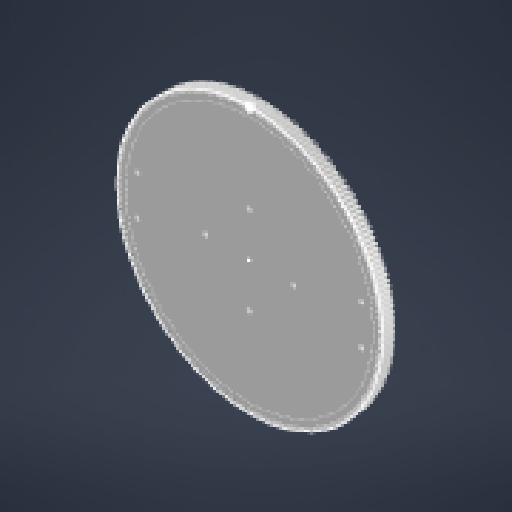
# Autodesk Inventor part: vertical_axis_bigl_gear
Saved by Autodesk Inventor 2023.2 (Build 272271000, 271)
## iProperties
Created: 2020-10-03
Part Number: vertical_axis_bigl_gear
Material: Generic
Document SubType Name: Modeling
Designer: bober
Density: 1 g/cm^3
Appearance: Default
Author: bober
Autodesk Inventor part; units mm, degrees
ref_plane "YZ Plane" through (0, 0, 0) normal (1, 0, 0) x (0, 1, 0)
ref_plane "XZ Plane" through (0, 0, 0) normal (0, 1, 0) x (-1, 0, 0)
ref_plane "XY Plane" through (0, 0, 0) normal (0, 0, 1) x (1, 0, 0)
sketch "Sketch1" plane through (0, 0, 0) normal (0, 0, 1) x (1, 0, 0)
  spline S0 degree 3 poles (-1.2656, 100.9921) (-1.1744, 100.7653) (-0.9921, 100.3117) (-0.7787, 99.7392) (-0.6166, 99.278) (-0.5147, 98.9901) (-0.458, 98.7994) (-0.4209, 98.7155) (-0.3986, 98.6754) (-0.3711, 98.6386) (-0.3402, 98.6046) (-0.3051, 98.575) (-0.267, 98.5494) (-0.2257, 98.5291) (-0.1823, 98.5143) (-0.1375, 98.5042) (-0.0764, 98.5001) (0, 98.5024) (0.0764, 98.5001) (0.1375, 98.5042) (0.1823, 98.5143) (0.2257, 98.5291) (0.267, 98.5494) (0.3051, 98.575) (0.3402, 98.6046) (0.3711, 98.6386) (0.3986, 98.6754) (0.4209, 98.7155) (0.458, 98.7994) (0.5147, 98.9901) (0.6166, 99.278) (0.7787, 99.7392) (0.9921, 100.3117) (1.1744, 100.7653) (1.2656, 100.9921) knots 0 0 0 0 0.07332 0.14664 0.1833 0.219961 0.238288 0.242867 0.247449 0.252032 0.256612 0.261194 0.265775 0.270356 0.274938 0.279519 0.284099 0.293264 0.30243 0.307009 0.311591 0.316173 0.320754 0.325335 0.329917 0.334497 0.33908 0.343662 0.348241 0.366568 0.403229 0.439889 0.513209 0.586529 0.586529 0.586529 0.586529
  circle A0 centre (0, 0) radius 98.5015 construction
  circle A1 centre (0, 0) radius 93.9693 construction
  circle A2 centre (0, 0) radius 100 construction
  circle A3 centre (0, 0) radius 101
  point P0 (-0.995, 100.3106)
  point P1 (-0.7389, 99.6236)
  point P2 (-0.6165, 99.2781)
  point P3 (-0.4982, 98.931)
  point P4 (-0.4391, 98.7576)
  point P5 (-0.4203, 98.7158)
  point P6 (-0.3977, 98.6759)
  point P7 (-0.3705, 98.6391)
  point P8 (-0.3395, 98.6053)
  point P9 (-0.3046, 98.5756)
  point P10 (-0.2665, 98.5503)
  point P11 (-0.2254, 98.53)
  point P12 (-0.1821, 98.5151)
  point P13 (-0.1373, 98.5053)
  point P14 (-0.0917, 98.5016)
  point P15 (0, 98.5015)
  point P16 (0.0917, 98.5016)
  point P17 (0.1373, 98.5053)
  point P18 (0.1821, 98.5151)
  point P19 (0.2254, 98.53)
  point P20 (0.2665, 98.5503)
  point P21 (0.3046, 98.5756)
  point P22 (0.3395, 98.6053)
  point P23 (0.3705, 98.6391)
  point P24 (0.3977, 98.6759)
  point P25 (0.4203, 98.7158)
  point P26 (0.4391, 98.7576)
  point P27 (0.4982, 98.931)
  point P28 (0.6165, 99.2781)
  point P29 (0.7389, 99.6236)
  point P30 (0.995, 100.3106)
  constraints: 4 centre point, 2 point on circle, 71 other
extrude "Extrusion1" add sketch "Sketch1" against normal blind 10
extrude "Extrusion2" cut sketch "Sketch1" against normal blind 10 contours A3 S0 picked at (-0.0238, 99.8482)
pattern_circular "Circular Pattern1" count 200 over 360 about axis through (0, 0, 0) along (0, 0, -1) of "Extrusion2"
sketch "Sketch20" plane through (0, 0, 0) normal (0, 0, 1) x (1, 0, 0)
  line L0 (-85, 20) -> (-85, -20) projected
  circle A0 centre (-85, -15) radius 2
  circle A1 centre (-85, 15) radius 2
  point P0 (0, 0)
  dimension "d80" = 4
  dimension "d81" = 4
  constraints: 2 centre point, 1 point on line
  measures "d80" diameter of A0
  measures "d81" diameter of A1
extrude "Extrusion14" cut sketch "Sketch20" against normal blind 10
sketch "Sketch21" plane through (0, 0, 0) normal (0, 0, 1) x (1, 0, 0)
  line L0 (85, -20) -> (85, 20) projected
  circle A0 centre (85, -15) radius 2
  circle A1 centre (85, 15) radius 2
  point P0 (0, 0)
  dimension "d84" = 4
  dimension "d85" = 4
  constraints: 2 centre point, 2 point on line
  measures "d84" diameter of A0
  measures "d85" diameter of A1
extrude "Extrusion15" cut sketch "Sketch21" against normal blind 10
sketch "Sketch29" plane through (0, 0, 0) normal (0, 0, 1) x (1, 0, 0)
  circle A0 centre (33.5, 0) radius 2
  circle A1 centre (-33.5, 0) radius 2
  circle A2 centre (0, 33.5) radius 2
  circle A3 centre (0, -33.5) radius 2
  point P0 (0, 0)
  dimension "d116" = 4
  dimension "d120" = 4
  dimension "d124" = 4
  dimension "d125" = 4
  constraints: 4 centre point
  measures "d116" diameter of A0
  measures "d120" diameter of A1
  measures "d124" diameter of A2
  measures "d125" diameter of A3
extrude "Extrusion23" cut sketch "Sketch29" against normal blind 10
sketch "Sketch30" plane through (0, 0, 0) normal (0, 0, 1) x (1, 0, 0)
  line L0 (135.3153, 25) -> (75, 25)
  line L1 (75, 25) -> (75, 10)
  line L2 (75, 10) -> (10, 10)
  line L3 (10, 10) -> (10, 43.5)
  line L4 (10, 43.5) -> (-0.1752, 43.5)
  line L5 (-0.1752, 43.5) -> (-0.1752, 120.9976)
  circle A0 centre (85, 15) radius 2 projected
  circle A1 centre (33.5, 0) radius 2 projected
  circle A2 centre (0, 33.5) radius 2 projected
  line L6 (-135.6656, 25) -> (-75.3503, 25)
  line L7 (-75.3503, 25) -> (-75.3503, 10)
  line L8 (-75.3503, 10) -> (-10.3503, 10)
  line L9 (-10.3503, 10) -> (-10.3503, 43.5)
  line L10 (-10.3503, 43.5) -> (-0.1752, 43.5)
  arc A3 (135.3153, 25) -> (-135.6656, 25) centre (-0.1752, 71.875) ccw
  arc A4 (-87.4986, -25) -> (-10, -90.4489) centre (0, 0) ccw
  circle A5 centre (0, 0) radius 101 projected
  line L11 (-10, -10) -> (-75, -10)
  line L12 (-75, -10) -> (-75, -25)
  circle A6 centre (0, -33.5) radius 2 projected
  circle A7 centre (-33.5, 0) radius 2 projected
  circle A8 centre (-85, -15) radius 2 projected
  line L13 (-10, -103.4371) -> (-10, -100.5037)
  line L14 (-10, -90.4489) -> (-10, -10)
  line L15 (-75, -25) -> (-87.4986, -25)
  line L16 (-97.857, -25) -> (-99.3218, -25)
  arc A9 (9.6497, -90.4489) -> (87.1482, -25) centre (-0.3503, 0) ccw
  line L17 (9.6497, -10) -> (74.6497, -10)
  line L18 (74.6497, -10) -> (74.6497, -25)
  line L19 (9.6497, -90.4489) -> (9.6497, -10)
  line L20 (74.6497, -25) -> (87.1482, -25)
  dimension "d126" = 10
  dimension "d127" = 10
  dimension "d128" = 10
  dimension "d129" = 10
  dimension "d130" = 10
  dimension "d134" = 10
  dimension "d136" = 10
  dimension "d137" = 10
  constraints: 42 end point, 11 symmetric about line, 10 perpendicular, 8 point on circle, 3 centre point, 2 vertical, 1 coincident, 1 horizontal, 1 other
  measures "d126" distance from line of L0 A0.centre
  measures "d127" distance from line of L1 A0.centre
  measures "d128" distance from line of L2 A1.centre
  measures "d129" distance from line of L3 A2.centre
  measures "d130" distance from line of L4 A2.centre
  measures "d134" radial gap between concentric circles of A4 A5
  measures "d136" distance from line of A7.centre L11
  measures "d137" distance from line of L12 A8.centre
extrude "Extrusion24" cut sketch "Sketch30" against normal through all contours L0 A5 L6 A3 | L0 L1 L2 L3 L4 L5 A5 | L5 L10 L9 L8 L7 L6 A5 | L15 L12 L11 L14 A4 | L19 L17 L18 L20 A9
sketch "Sketch31" plane through (0, 0, 0) normal (0, 0, 1) x (1, 0, 0)
  circle A0 centre (0, 0) radius 100 construction
  circle A1 centre (0, 0) radius 100
  constraints: 1 centre point, 1 coincident, 1 concentric
surface extrude "ExtrusionSrf1" sketch "Sketch31" against normal up to surface (10 mm away) shown yes curves A1
equation "\"d0\" = FaceWidth"
equation "\"Module\" = 1"
equation "\"PressureAngle\" = 20deg"
equation "\"UnitProfileClearance\" = 0.25"
equation "\"UnitRoundRadius\" = 0.35"
equation "\"HeadDiameter\" = 202"
equation "\"RootDiameter\" = 197.00295"
equation "\"BaseDiameter\" = 187.93852"
equation "\"FaceWidth\" = 10"
equation "\"HelixAngle\" = 0"
equation "\"UnitCorrection\" = 0"
equation "\"UnitAddendumModification\" = 0"
equation "\"CircularPitch\" = 3.141593"
equation "\"UnitBacklashShift\" = -0.248523"
equation "\"TotalToolShift\" = -0.24852"
equation "\"IsInternal\" = 0"
body "Solid1"
body "Srf1"
